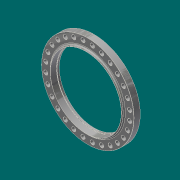
# Autodesk Inventor part: A1-19027-200-xx 30in CL250 flange
Saved by Autodesk Inventor 2017.3 (Build 213256000, 256)
## iProperties
Created: 2019-06-26
Part Number: A1-19027-200-xx 30in CL250 flange
Material: Steel, Mild
Document SubType Name: Modeling
Designer: Graeme_Van_Dongen
Density: 7.85 g/cm^3
Appearance: Steel
Author: Graeme_Van_Dongen
Autodesk Inventor part; units mm, degrees
ref_plane "YZ Plane" through (0, 0, 0) normal (1, 0, 0) x (0, 1, 0)
ref_plane "XZ Plane" through (0, 0, 0) normal (0, 1, 0) x (-1, 0, 0)
sketch "Sketch1" plane through (0, 0, 0) normal (0, 0, 1) x (1, 0, 0)
  circle A0 centre (0, 0) radius 546.1
  dimension "d0" = 1092.2
  constraints: 1 centre point, 1 coincident
  measures "d0" diameter of A0
extrude "Extrusion1" add sketch "Sketch1" along normal blind 76.2
sketch "Sketch2" plane through (0, 0, 76.2) normal (0, 0, 1) x (1, 0, 0)
  line L0 (-55.8115, -495.3407) -> (55.8115, 495.3407) construction
  line L1 (0, -764.54) -> (0, 764.54) construction
  point P0 (0, 0)
  point P1 (0, 0)
  dimension "d3" = 996.95
  dimension "d4" = 6.429
  constraints: 2 coincident, 2 end point, 1 midpoint
  measures "d3" distance of L0.start L0.end
  measures "d4" angle of L0 L1
hole "Hole1" at (55.8115, 495.3407, 76.2) direction (0, 0, -1) diameter 47.625 end through all
chamfer "Chamfer1" distance 1.5875 angle 45 2 edges at (55.8115, 519.1532, 76.2) (55.8115, 519.1532, 0)
pattern_circular "Circular Pattern1" count 28 over 360 about axis through (0, 0, -10) along (0, 0, 1) of "Hole1", "Chamfer1"
chamfer "Chamfer2" distance 1.5875 angle 45 2 edges at (-546.1, 0, 76.2) (-546.1, 0, 0)
sketch "Sketch3" plane through (0, 0, 76.2) normal (0, 0, 1) x (1, 0, 0)
  circle A0 centre (0, 0) radius 447.675
  dimension "d21" = 895.35
  constraints: 1 centre point, 1 coincident
  measures "d21" diameter of A0
ref_plane "Work Plane1" through (0, 0, 152.4) normal (0, 0, 1) x (1, 0, 0)
sketch "Sketch4" plane through (0, 0, 152.4) normal (0, 0, 1) x (1, 0, 0)
  circle A0 centre (0, 0) radius 381
  dimension "d23" = 762
  constraints: 1 centre point, 1 coincident
  measures "d23" diameter of A0
extrude "Extrusion2" add sketch "Sketch4" against normal blind 12.7
loft "Loft1" add profiles "Sketch3" section 1 edges at (-381, 0, 139.7)
fillet "Fillet1" radius 12.7 1 edges at (-447.675, 0, 76.2)
sketch "Sketch5" plane through (0, 0, 0) normal (1, 0, 0) x (0, 1, 0)
  line L0 (443.9964, 79.7034) -> (381, 139.7) construction
  arc A0 (443.9964, 79.7034) -> (452.755, 76.2) centre (452.755, 88.9) ccw construction
  line L1 (381, 152.4) -> (381, 139.7) construction
  line L2 (0, -30.48) -> (0, 182.88) projected
  line L3 (0, 0) -> (419.1, 0)
  line L4 (419.1, 0) -> (419.1, 98.425)
  line L5 (419.1, 98.425) -> (420.6875, 98.425)
  line L6 (420.6875, 98.425) -> (431.8, 89.8981)
  line L7 (431.8, 89.8981) -> (431.8, 88.9)
  arc A1 (431.8, 88.9) -> (444.5, 76.2) centre (444.5, 88.9) ccw
  line L8 (444.5, 76.2) -> (452.755, 76.2)
  line L9 (452.755, 76.2) -> (452.755, 152.4)
  line L10 (452.755, 152.4) -> (0, 152.4)
  dimension "d31" = 863.6
  dimension "d32" = 12.7
  dimension "d33" = 11.1125
  dimension "d34" = 37.5
  dimension "d35" = 12.7
  dimension "d36" = 98.425
  dimension "d37" = 0.9981
  constraints: 16 end point, 3 perpendicular, 2 horizontal, 2 point on circle, 2 point on line, 2 tangent, 1 centre point, 1 parallel, 1 vertical
  measures "d31" diameter of L7 L2
  measures "d32" distance between parallel lines of L4 L7
  measures "d33" horizontal distance of L5.end L6.end
  measures "d34" angle of L5 L6
  measures "d35" radius of A1
  measures "d36" distance between parallel lines of L3 L5
  measures "d37" distance of L6.end L7.end
revolve "Revolution1" cut sketch "Sketch5" angle 360 about axis through (0, 0, -10) along (0, 0, 1)
sketch "Sketch6" plane through (0, 0, 0) normal (0, 0, -1) x (-1, 0, 0)
  circle A0 centre (0, 0) radius 419.1 projected
  circle A1 centre (0, 0) radius 412.75
  dimension "d39" = 825.5
  constraints: 1 centre point, 1 coincident
  measures "d39" diameter of A1
extrude "Extrusion3" add sketch "Sketch6" against normal blind 25.4
chamfer "Chamfer3" distance 0.7937 angle 45 1 edges at (412.75, 0, 25.4)
fillet "Fillet2" radius 0.7937 1 edges at (0, -419.1, 25.4)
body "Solid1"
